Autodesk Fusion 360 part; units mm, degrees
(part 2 of 4)
extrude "Extrusion32" add sketch "Skizze34" along normal blind 12 contours L15 L31 L36 L66 L67 L68 L69 bodies 2
sketch "Skizze35" plane through (0, 47, 0) normal (0, 1, 0) x (-1, 0, 0)
  line L0 (23, -18.5) -> (23, -10.5)
  line L1 (23, -10.5) -> (30, -10.5)
  line L2 (30, -10.5) -> (30, -18.5)
  line L3 (30, -18.5) -> (23, -18.5)
  line L4 (21.5, -1.5) -> (21.5, -23.5)
  line L5 (21.5, -23.5) -> (-5.5, -23.5)
  line L6 (-5.5, -23.5) -> (-5.5, -1.5)
  line L7 (-5.5, -1.5) -> (21.5, -1.5)
  circle A0 centre (36, -25) radius 1.9
  circle A1 centre (-36, -14.5) radius 1.9
  circle A2 centre (36, 25) radius 1.9
  circle A3 centre (-36, 14.5) radius 1.9
  line L8 (-12, 21.5) -> (-12, 11.5)
  line L9 (-12, 11.5) -> (-21, 11.5)
  line L10 (-21, 11.5) -> (-21, 21.5)
  line L11 (-21, 21.5) -> (-22.5, 21.5)
  line L12 (-22.5, 21.5) -> (-22.5, 27.5)
  line L13 (-22.5, 27.5) -> (-32.5, 27.5)
  line L14 (-32.5, 27.5) -> (-32.5, 19)
  arc A4 (-33.5, 18) -> (-32.5, 19) centre (-33.5, 19) ccw
  line L15 (-33.5, 18) -> (-38.5, 18)
  arc A5 (-38.5, 18) -> (-39.5, 17) centre (-38.5, 17) ccw
  line L16 (-39.5, 17) -> (-39.5, 12)
  arc A6 (-40.5, 11) -> (-39.5, 12) centre (-40.5, 12) ccw
  line L17 (-40.5, 11) -> (-56.5, 11)
  line L18 (-56.5, 11) -> (-56.5, -11)
  line L19 (-56.5, -11) -> (-40.5, -11)
  arc A7 (-39.5, -12) -> (-40.5, -11) centre (-40.5, -12) ccw
  line L20 (-39.5, -12) -> (-39.5, -17)
  arc A8 (-39.5, -17) -> (-38.5, -18) centre (-38.5, -17) ccw
  line L21 (-38.5, -18) -> (-33.5, -18)
  arc A9 (-32.5, -19) -> (-33.5, -18) centre (-33.5, -19) ccw
  line L22 (-32.5, -19) -> (-32.5, -27.5)
  line L23 (-32.5, -27.5) -> (32.5, -27.5)
  line L24 (32.5, -27.5) -> (34.8649, -28.3108)
  arc A10 (34.8649, -28.3108) -> (38.922, -26.9266) centre (36, -25) ccw
  line L25 (38.922, -26.9266) -> (42.5, -21.5)
  line L26 (42.5, -21.5) -> (57.5, -6.5)
  line L27 (57.5, -6.5) -> (57.5, 6.5)
  line L28 (57.5, 6.5) -> (42.5, 21.5)
  line L29 (42.5, 21.5) -> (38.922, 26.9266)
  arc A11 (38.922, 26.9266) -> (34.8649, 28.3108) centre (36, 25) ccw
  line L30 (34.8649, 28.3108) -> (32.5, 27.5)
  line L31 (32.5, 27.5) -> (-10.5, 27.5)
  line L32 (-10.5, 27.5) -> (-10.5, 21.5)
  line L33 (-10.5, 21.5) -> (-12, 21.5)
  circle A12 centre (3.5, 16) radius 6.5
  line L34 (-1.75, 0) -> (-22.5, 0)
  line L35 (45, 1.5) -> (34, 1.5)
  arc A13 (34, 1.5) -> (34, -1.5) centre (34, 0) ccw
  line L36 (34, -1.5) -> (45, -1.5)
  arc A14 (45, -1.5) -> (45, 1.5) centre (45, 0) ccw
  line L37 (45, 0) -> (34, 0) construction
  arc A15 (45, -13.5) -> (45, -10.5) centre (45, -12) ccw
  line L38 (34, -13.5) -> (45, -13.5)
  arc A16 (34, -10.5) -> (34, -13.5) centre (34, -12) ccw
  line L39 (45, -10.5) -> (34, -10.5)
  arc A17 (45, -7.5) -> (45, -4.5) centre (45, -6) ccw
  line L40 (34, -7.5) -> (45, -7.5)
  arc A18 (34, -4.5) -> (34, -7.5) centre (34, -6) ccw
  line L41 (45, -4.5) -> (34, -4.5)
  arc A19 (45, 4.5) -> (45, 7.5) centre (45, 6) ccw
  line L42 (34, 4.5) -> (45, 4.5)
  arc A20 (34, 7.5) -> (34, 4.5) centre (34, 6) ccw
  line L43 (45, 7.5) -> (34, 7.5)
  arc A21 (45, 10.5) -> (45, 13.5) centre (45, 12) ccw
  line L44 (34, 10.5) -> (45, 10.5)
  arc A22 (34, 13.5) -> (34, 10.5) centre (34, 12) ccw
  line L45 (45, 13.5) -> (34, 13.5)
  line L46 (-48.5, -1.5) -> (-37.3325, -1.5)
  arc A23 (-37.3325, -1.5) -> (-37.3325, 1.5) centre (-37.3325, 0) ccw
  line L47 (-37.3325, 1.5) -> (-48.5, 1.5)
  arc A24 (-48.5, 1.5) -> (-48.5, -1.5) centre (-48.5, 0) ccw
  line L48 (-48.5, 0) -> (-37.3325, 0) construction
  arc A25 (-37.3325, -7.5) -> (-37.3325, -4.5) centre (-37.3325, -6) ccw
  line L49 (-48.5, -7.5) -> (-37.3325, -7.5)
  line L50 (-37.3325, -4.5) -> (-48.5, -4.5)
  arc A26 (-48.5, -4.5) -> (-48.5, -7.5) centre (-48.5, -6) ccw
  arc A27 (-37.3325, 4.5) -> (-37.3325, 7.5) centre (-37.3325, 6) ccw
  line L51 (-48.5, 4.5) -> (-37.3325, 4.5)
  line L52 (-37.3325, 7.5) -> (-48.5, 7.5)
  arc A28 (-48.5, 7.5) -> (-48.5, 4.5) centre (-48.5, 6) ccw
  line L53 (-12.5, 8.9343) -> (-20.5, 8.9343)
  arc A29 (-20.5, 8.9343) -> (-20.5, 6.9343) centre (-20.5, 7.9343) ccw
  line L54 (-20.5, 6.9343) -> (-12.5, 6.9343)
  arc A30 (-12.5, 6.9343) -> (-12.5, 8.9343) centre (-12.5, 7.9343) ccw
  line L55 (-12.5, 7.9343) -> (-20.5, 7.9343) construction
  arc A31 (-12.5, 2.5057) -> (-12.5, 4.5057) centre (-12.5, 3.5057) ccw
  line L56 (-20.5, 2.5057) -> (-12.5, 2.5057)
  line L57 (-12.5, 4.5057) -> (-20.5, 4.5057)
  arc A32 (-20.5, 4.5057) -> (-20.5, 2.5057) centre (-20.5, 3.5057) ccw
  arc A33 (-12.5, -1.9228) -> (-12.5, 0.0772) centre (-12.5, -0.9228) ccw
  line L58 (-20.5, -1.9228) -> (-12.5, -1.9228)
  line L59 (-12.5, 0.0772) -> (-20.5, 0.0772)
  arc A34 (-20.5, 0.0772) -> (-20.5, -1.9228) centre (-20.5, -0.9228) ccw
  arc A35 (-12.5, -6.3514) -> (-12.5, -4.3514) centre (-12.5, -5.3514) ccw
  line L60 (-20.5, -6.3514) -> (-12.5, -6.3514)
  line L61 (-12.5, -4.3514) -> (-20.5, -4.3514)
  arc A36 (-20.5, -4.3514) -> (-20.5, -6.3514) centre (-20.5, -5.3514) ccw
  arc A37 (-12.5, -10.78) -> (-12.5, -8.78) centre (-12.5, -9.78) ccw
  line L62 (-20.5, -10.78) -> (-12.5, -10.78)
  line L63 (-12.5, -8.78) -> (-20.5, -8.78)
  arc A38 (-20.5, -8.78) -> (-20.5, -10.78) centre (-20.5, -9.78) ccw
  arc A39 (-12.5, -15.2086) -> (-12.5, -13.2086) centre (-12.5, -14.2086) ccw
  line L64 (-20.5, -15.2086) -> (-12.5, -15.2086)
  line L65 (-12.5, -13.2086) -> (-20.5, -13.2086)
  arc A40 (-20.5, -13.2086) -> (-20.5, -15.2086) centre (-20.5, -14.2086) ccw
  arc A41 (-12.5, -19.6371) -> (-12.5, -17.6371) centre (-12.5, -18.6371) ccw
  line L66 (-20.5, -19.6371) -> (-12.5, -19.6371)
  line L67 (-12.5, -17.6371) -> (-20.5, -17.6371)
  arc A42 (-20.5, -17.6371) -> (-20.5, -19.6371) centre (-20.5, -18.6371) ccw
  arc A43 (-12.5, -24.0657) -> (-12.5, -22.0657) centre (-12.5, -23.0657) ccw
  line L68 (-20.5, -24.0657) -> (-12.5, -24.0657)
  line L69 (-12.5, -22.0657) -> (-20.5, -22.0657)
  arc A44 (-20.5, -22.0657) -> (-20.5, -24.0657) centre (-20.5, -23.0657) ccw
  dimension "d166" = 3
  dimension "d169" = 0
  dimension "d170" = 12
  dimension "d171" = 3
  dimension "d174" = 0
  dimension "d175" = 6
  dimension "d176" = 2
  dimension "d179" = 0
  dimension "d180" = -31
  measures "d166" diameter of A13
  measures "d171" diameter of A23
  measures "d176" diameter of A29
extrude "Extrusion33" cut sketch "Skizze35" against normal blind 2 contours L34 A33 L58 A34 | L35 A13 L36 A14 | A15 L38 A16 L39 | A17 L40 A18 L41 | A19 L42 A20 L43 | A21 L44 A22 L45 | L46 A23 L47 A24 | A25 L49 L50 A26 | A27 L51 L52 A28 | L53 A29 L54 A30 | A31 L56 L57 A32 | A35 L60 L61 A36 | A37 L62 L63 A38 | A39 L64 L65 A40 | A41 L66 L67 A42 | A43 L68 L69 A44 bodies 2
sketch "Skizze37" plane through (0, 45, 0) normal (0, -1, 0) x (1, 0, 0)
  line L0 (48.5, -7.5) -> (37.3325, -7.5)
  arc A0 (37.3325, -4.5) -> (37.3325, -7.5) centre (37.3325, -6) ccw
  line L1 (37.3325, -4.5) -> (48.5, -4.5)
  arc A1 (48.5, -7.5) -> (48.5, -4.5) centre (48.5, -6) ccw
  line L2 (20.5, -6.3514) -> (12.5, -6.3514)
  arc A2 (12.5, -4.3514) -> (12.5, -6.3514) centre (12.5, -5.3514) ccw
  line L3 (12.5, -4.3514) -> (20.5, -4.3514)
  arc A3 (20.5, -6.3514) -> (20.5, -4.3514) centre (20.5, -5.3514) ccw
  line L4 (20.5, -24.0657) -> (12.5, -24.0657)
  arc A4 (12.5, -22.0657) -> (12.5, -24.0657) centre (12.5, -23.0657) ccw
  line L5 (12.5, -22.0657) -> (20.5, -22.0657)
  arc A5 (20.5, -24.0657) -> (20.5, -22.0657) centre (20.5, -23.0657) ccw
  arc A6 (-34, -7.5) -> (-34, -4.5) centre (-34, -6) ccw
  line L6 (-34, -7.5) -> (-45, -7.5)
  arc A7 (-45, -4.5) -> (-45, -7.5) centre (-45, -6) ccw
  line L7 (-45, -4.5) -> (-34, -4.5)
  line L8 (-45, 1.5) -> (-34, 1.5)
  arc A8 (-34, -1.5) -> (-34, 1.5) centre (-34, 0) ccw
  line L9 (-34, -1.5) -> (-45, -1.5)
  arc A9 (-45, 1.5) -> (-45, -1.5) centre (-45, 0) ccw
  line L10 (20.5, -19.6371) -> (12.5, -19.6371)
  arc A10 (12.5, -17.6371) -> (12.5, -19.6371) centre (12.5, -18.6371) ccw
  line L11 (12.5, -17.6371) -> (20.5, -17.6371)
  arc A11 (20.5, -19.6371) -> (20.5, -17.6371) centre (20.5, -18.6371) ccw
  arc A12 (20.5, -1.9228) -> (20.8852, 0) centre (20.5, -0.9228) ccw
  line L12 (20.5, -1.9228) -> (12.5, -1.9228)
  arc A13 (12.1148, 0) -> (12.5, -1.9228) centre (12.5, -0.9228) ccw
  line L13 (12.1148, 0) -> (20.8852, 0)
  line L14 (48.5, -1.5) -> (37.3325, -1.5)
  arc A14 (37.3325, 1.5) -> (37.3325, -1.5) centre (37.3325, 0) ccw
  line L15 (37.3325, 1.5) -> (48.5, 1.5)
  arc A15 (48.5, -1.5) -> (48.5, 1.5) centre (48.5, 0) ccw
  line L16 (12.5, 8.9343) -> (20.5, 8.9343)
  arc A16 (20.5, 6.9343) -> (20.5, 8.9343) centre (20.5, 7.9343) ccw
  line L17 (20.5, 6.9343) -> (12.5, 6.9343)
  arc A17 (12.5, 8.9343) -> (12.5, 6.9343) centre (12.5, 7.9343) ccw
  line L18 (20.5, -10.78) -> (12.5, -10.78)
  arc A18 (12.5, -8.78) -> (12.5, -10.78) centre (12.5, -9.78) ccw
  line L19 (12.5, -8.78) -> (20.5, -8.78)
  arc A19 (20.5, -10.78) -> (20.5, -8.78) centre (20.5, -9.78) ccw
  arc A20 (-34, 10.5) -> (-34, 13.5) centre (-34, 12) ccw
  line L20 (-34, 10.5) -> (-45, 10.5)
  arc A21 (-45, 13.5) -> (-45, 10.5) centre (-45, 12) ccw
  line L21 (-45, 13.5) -> (-34, 13.5)
  arc A22 (-34, -13.5) -> (-34, -10.5) centre (-34, -12) ccw
  line L22 (-34, -13.5) -> (-45, -13.5)
  arc A23 (-45, -10.5) -> (-45, -13.5) centre (-45, -12) ccw
  line L23 (-45, -10.5) -> (-34, -10.5)
  arc A24 (-34, 4.5) -> (-34, 7.5) centre (-34, 6) ccw
  line L24 (-34, 4.5) -> (-45, 4.5)
  arc A25 (-45, 7.5) -> (-45, 4.5) centre (-45, 6) ccw
  line L25 (-45, 7.5) -> (-34, 7.5)
  line L26 (20.5, -15.2086) -> (12.5, -15.2086)
  arc A26 (12.5, -13.2086) -> (12.5, -15.2086) centre (12.5, -14.2086) ccw
  line L27 (12.5, -13.2086) -> (20.5, -13.2086)
  arc A27 (20.5, -15.2086) -> (20.5, -13.2086) centre (20.5, -14.2086) ccw
  line L28 (20.5, 2.5057) -> (12.5, 2.5057)
  arc A28 (12.5, 4.5057) -> (12.5, 2.5057) centre (12.5, 3.5057) ccw
  line L29 (12.5, 4.5057) -> (20.5, 4.5057)
  arc A29 (20.5, 2.5057) -> (20.5, 4.5057) centre (20.5, 3.5057) ccw
  line L30 (48.5, 4.5) -> (37.3325, 4.5)
  arc A30 (37.3325, 7.5) -> (37.3325, 4.5) centre (37.3325, 6) ccw
  line L31 (37.3325, 7.5) -> (48.5, 7.5)
  arc A31 (48.5, 4.5) -> (48.5, 7.5) centre (48.5, 6) ccw
  line L32 (-21.5, -20) -> (-31, -20)
  line L33 (-31, -20) -> (-31, -26)
  line L34 (-31, -26) -> (-23, -26)
  line L35 (-23, -26) -> (23, -26)
  line L36 (23, -26) -> (31, -26)
  line L37 (31, -26) -> (31, -9.5)
  line L38 (31, -9.5) -> (51.5, -9.5)
  line L39 (51.5, -9.5) -> (51.5, 9.5)
  line L40 (51.5, 9.5) -> (31, 9.5)
  line L41 (31, 9.5) -> (31, 26)
  line L42 (31, 26) -> (22.5, 26)
  line L43 (22.5, 26) -> (22.5, 21.5)
  line L44 (22.5, 21.5) -> (21, 21.5)
  line L45 (21, 21.5) -> (21, 11.5)
  line L46 (21, 11.5) -> (12, 11.5)
  line L47 (12, 11.5) -> (12, 21.5)
  line L48 (12, 21.5) -> (10.5, 21.5)
  line L49 (10.5, 21.5) -> (10.5, 26)
  line L50 (10.5, 26) -> (-31, 26)
  line L51 (-31, 26) -> (-31, 20)
  line L52 (-31, 20) -> (-41.8787, 20)
  line L53 (-41.8787, 20) -> (-51.5218, 10.3569)
  line L54 (-51.5218, 10.3569) -> (-51.5218, -10.3569)
  line L55 (-51.5218, -10.3569) -> (-41.8787, -20)
  line L56 (-41.8787, -20) -> (-31.5, -20)
  line L57 (-31.5, -20) -> (-31.5, -9)
  line L58 (-31.5, -9) -> (-21.5, -9)
  line L59 (-21.5, -9) -> (-21.5, -4.5)
  line L60 (-21.5, -4.5) -> (5.5, -4.5)
  line L61 (5.5, -4.5) -> (5.5, -20.5)
  line L62 (5.5, -20.5) -> (-21.5, -20.5)
  line L63 (-21.5, -20.5) -> (-21.5, -20)
  circle A32 centre (-3.5, 16) radius 6.5
  line L64 (26, -25.5) -> (8, -25.5)
  line L65 (8, -25.5) -> (8, 10.5)
  line L66 (8, 10.5) -> (26, 10.5)
  line L67 (26, 10.5) -> (26, -25.5)
  dimension "d185" = 18
  dimension "d186" = 36
  dimension "d187" = 8
  dimension "d188" = 5
  dimension "d189" = 1
  measures "d185" distance of origin
  measures "d186" distance of origin
  measures "d188" distance of L45 L67
  measures "d189" distance of L46 L66
extrude "Extrusion35" cut sketch "Skizze37" against normal blind 1 contours L64 L65 L66 L67 bodies 2
sketch "Skizze38" plane through (0, 47, 0) normal (0, 1, 0) x (-1, 0, 0)
  line L0 (-37.3325, -7.5) -> (-48.5, -7.5)
  arc A0 (-48.5, -4.5) -> (-48.5, -7.5) centre (-48.5, -6) ccw
  line L1 (-48.5, -4.5) -> (-37.3325, -4.5)
  arc A1 (-37.3325, -7.5) -> (-37.3325, -4.5) centre (-37.3325, -6) ccw
  line L2 (-12.5, -6.3514) -> (-20.5, -6.3514)
  arc A2 (-20.5, -4.3514) -> (-20.5, -6.3514) centre (-20.5, -5.3514) ccw
  line L3 (-20.5, -4.3514) -> (-12.5, -4.3514)
  arc A3 (-12.5, -6.3514) -> (-12.5, -4.3514) centre (-12.5, -5.3514) ccw
  line L4 (-12.5, -24.0657) -> (-20.5, -24.0657)
  arc A4 (-20.5, -22.0657) -> (-20.5, -24.0657) centre (-20.5, -23.0657) ccw
  line L5 (-20.5, -22.0657) -> (-12.5, -22.0657)
  arc A5 (-12.5, -24.0657) -> (-12.5, -22.0657) centre (-12.5, -23.0657) ccw
  arc A6 (34, -4.5) -> (34, -7.5) centre (34, -6) ccw
  line L6 (34, -4.5) -> (45, -4.5)
  arc A7 (45, -7.5) -> (45, -4.5) centre (45, -6) ccw
  line L7 (45, -7.5) -> (34, -7.5)
  line L8 (34, 1.5) -> (45, 1.5)
  arc A8 (45, -1.5) -> (45, 1.5) centre (45, 0) ccw
  line L9 (45, -1.5) -> (34, -1.5)
  arc A9 (34, 1.5) -> (34, -1.5) centre (34, 0) ccw
  line L10 (-12.5, -19.6371) -> (-20.5, -19.6371)
  arc A10 (-20.5, -17.6371) -> (-20.5, -19.6371) centre (-20.5, -18.6371) ccw
  line L11 (-20.5, -17.6371) -> (-12.5, -17.6371)
  arc A11 (-12.5, -19.6371) -> (-12.5, -17.6371) centre (-12.5, -18.6371) ccw
  arc A12 (-20.8852, 0) -> (-20.5, -1.9228) centre (-20.5, -0.9228) ccw
  line L12 (-20.8852, 0) -> (-12.1148, 0)
  arc A13 (-12.5, -1.9228) -> (-12.1148, 0) centre (-12.5, -0.9228) ccw
  line L13 (-12.5, -1.9228) -> (-20.5, -1.9228)
  line L14 (-37.3325, -1.5) -> (-48.5, -1.5)
  arc A14 (-48.5, 1.5) -> (-48.5, -1.5) centre (-48.5, 0) ccw
  line L15 (-48.5, 1.5) -> (-37.3325, 1.5)
  arc A15 (-37.3325, -1.5) -> (-37.3325, 1.5) centre (-37.3325, 0) ccw
  line L16 (-20.5, 8.9343) -> (-12.5, 8.9343)
  arc A16 (-12.5, 6.9343) -> (-12.5, 8.9343) centre (-12.5, 7.9343) ccw
  line L17 (-12.5, 6.9343) -> (-20.5, 6.9343)
  arc A17 (-20.5, 8.9343) -> (-20.5, 6.9343) centre (-20.5, 7.9343) ccw
  line L18 (-12.5, -10.78) -> (-20.5, -10.78)
  arc A18 (-20.5, -8.78) -> (-20.5, -10.78) centre (-20.5, -9.78) ccw
  line L19 (-20.5, -8.78) -> (-12.5, -8.78)
  arc A19 (-12.5, -10.78) -> (-12.5, -8.78) centre (-12.5, -9.78) ccw
  arc A20 (34, 13.5) -> (34, 10.5) centre (34, 12) ccw
  line L20 (34, 13.5) -> (45, 13.5)
  arc A21 (45, 10.5) -> (45, 13.5) centre (45, 12) ccw
  line L21 (45, 10.5) -> (34, 10.5)
  arc A22 (34, -10.5) -> (34, -13.5) centre (34, -12) ccw
  line L22 (34, -10.5) -> (45, -10.5)
  arc A23 (45, -13.5) -> (45, -10.5) centre (45, -12) ccw
  line L23 (45, -13.5) -> (34, -13.5)
  arc A24 (34, 7.5) -> (34, 4.5) centre (34, 6) ccw
  line L24 (34, 7.5) -> (45, 7.5)
  arc A25 (45, 4.5) -> (45, 7.5) centre (45, 6) ccw
  line L25 (45, 4.5) -> (34, 4.5)
  line L26 (-12.5, -15.2086) -> (-20.5, -15.2086)
  arc A26 (-20.5, -13.2086) -> (-20.5, -15.2086) centre (-20.5, -14.2086) ccw
  line L27 (-20.5, -13.2086) -> (-12.5, -13.2086)
  arc A27 (-12.5, -15.2086) -> (-12.5, -13.2086) centre (-12.5, -14.2086) ccw
  line L28 (-12.5, 2.5057) -> (-20.5, 2.5057)
  arc A28 (-20.5, 4.5057) -> (-20.5, 2.5057) centre (-20.5, 3.5057) ccw
  line L29 (-20.5, 4.5057) -> (-12.5, 4.5057)
  arc A29 (-12.5, 2.5057) -> (-12.5, 4.5057) centre (-12.5, 3.5057) ccw
  line L30 (-37.3325, 4.5) -> (-48.5, 4.5)
  arc A30 (-48.5, 7.5) -> (-48.5, 4.5) centre (-48.5, 6) ccw
  line L31 (-48.5, 7.5) -> (-37.3325, 7.5)
  arc A31 (-37.3325, 4.5) -> (-37.3325, 7.5) centre (-37.3325, 6) ccw
  line L32 (23, -18.5) -> (23, -10.5)
  line L33 (23, -10.5) -> (30, -10.5)
  line L34 (30, -10.5) -> (30, -18.5)
  line L35 (30, -18.5) -> (23, -18.5)
  line L36 (21.5, -1.5) -> (21.5, -23.5)
  line L37 (21.5, -23.5) -> (-5.5, -23.5)
  line L38 (-5.5, -23.5) -> (-5.5, -1.5)
  line L39 (-5.5, -1.5) -> (21.5, -1.5)
  circle A32 centre (-36, 14.5) radius 1.9
  circle A33 centre (36, 25) radius 1.9
  circle A34 centre (36, -25) radius 1.9
  circle A35 centre (-36, -14.5) radius 1.9
  line L40 (-12, 21.5) -> (-12, 11.5)
  line L41 (-12, 11.5) -> (-21, 11.5)
  line L42 (-21, 11.5) -> (-21, 21.5)
  line L43 (-21, 21.5) -> (-22.5, 21.5)
  line L44 (-22.5, 21.5) -> (-22.5, 27.5)
  line L45 (-22.5, 27.5) -> (-32.5, 27.5)
  line L46 (-32.5, 27.5) -> (-32.5, 19)
  arc A36 (-33.5, 18) -> (-32.5, 19) centre (-33.5, 19) ccw
  line L47 (-33.5, 18) -> (-38.5, 18)
  arc A37 (-38.5, 18) -> (-39.5, 17) centre (-38.5, 17) ccw
  line L48 (-39.5, 17) -> (-39.5, 12)
  arc A38 (-40.5, 11) -> (-39.5, 12) centre (-40.5, 12) ccw
  line L49 (-40.5, 11) -> (-56.5, 11)
  line L50 (-56.5, 11) -> (-56.5, -11)
  line L51 (-56.5, -11) -> (-40.5, -11)
  arc A39 (-39.5, -12) -> (-40.5, -11) centre (-40.5, -12) ccw
  line L52 (-39.5, -12) -> (-39.5, -17)
  arc A40 (-39.5, -17) -> (-38.5, -18) centre (-38.5, -17) ccw
  line L53 (-38.5, -18) -> (-33.5, -18)
  arc A41 (-32.5, -19) -> (-33.5, -18) centre (-33.5, -19) ccw
  line L54 (-32.5, -19) -> (-32.5, -27.5)
  line L55 (-32.5, -27.5) -> (32.5, -27.5)
  line L56 (32.5, -27.5) -> (34.8649, -28.3108)
  arc A42 (34.8649, -28.3108) -> (38.922, -26.9266) centre (36, -25) ccw
  line L57 (38.922, -26.9266) -> (42.5, -21.5)
  line L58 (42.5, -21.5) -> (57.5, -6.5)
  line L59 (57.5, -6.5) -> (57.5, 6.5)
  line L60 (57.5, 6.5) -> (42.5, 21.5)
  line L61 (42.5, 21.5) -> (38.922, 26.9266)
  arc A43 (38.922, 26.9266) -> (34.8649, 28.3108) centre (36, 25) ccw
  line L62 (34.8649, 28.3108) -> (32.5, 27.5)
  line L63 (32.5, 27.5) -> (-10.5, 27.5)
  line L64 (-10.5, 27.5) -> (-10.5, 21.5)
  line L65 (-10.5, 21.5) -> (-12, 21.5)
  circle A44 centre (3.5, 16) radius 6.5
  line L66 (23, -18.5) -> (22.3, -18.5)
  line L67 (22.3, -18.5) -> (22.3, -10.5)
  line L68 (22.3, -10.5) -> (23, -10.5)
  line L69 (23, -10.5) -> (23, -18.5)
  dimension "d192" = 0.7
  dimension "d194" = 0.8
  measures "d194" distance of L36 L67
extrude "Extrusion36" cut sketch "Skizze38" against normal blind 14 contours L32 L66 L67 L68 L69 bodies 2
sketch "Skizze39" plane through (0, 0, 0) normal (0, -1, 0) x (1, 0, 0)
  circle A0 centre (36, 14.5) radius 1.9
  circle A1 centre (36, -14.5) radius 1.9
  circle A2 centre (-36, -25) radius 1.9
  circle A3 centre (-36, 25) radius 1.9
  arc A4 (38.5, -18) -> (39.5, -17) centre (38.5, -17) ccw
  line L0 (39.5, -17) -> (39.5, -12)
  arc A5 (40.5, -11) -> (39.5, -12) centre (40.5, -12) ccw
  line L1 (40.5, -11) -> (56.5, -11)
  line L2 (56.5, -11) -> (56.5, 11)
  line L3 (56.5, 11) -> (40.5, 11)
  arc A6 (39.5, 12) -> (40.5, 11) centre (40.5, 12) ccw
  line L4 (39.5, 12) -> (39.5, 17)
  arc A7 (39.5, 17) -> (38.5, 18) centre (38.5, 17) ccw
  line L5 (38.5, 18) -> (33.5, 18)
  arc A8 (32.5, 19) -> (33.5, 18) centre (33.5, 19) ccw
  line L6 (32.5, 19) -> (32.5, 27.5)
  line L7 (32.5, 27.5) -> (-32.5, 27.5)
  line L8 (-32.5, 27.5) -> (-34.8649, 28.3108)
  arc A9 (-34.8649, 28.3108) -> (-38.922, 26.9266) centre (-36, 25) ccw
  line L9 (-38.922, 26.9266) -> (-42.5, 21.5)
  line L10 (-42.5, 21.5) -> (-57.5, 6.5)
  line L11 (-57.5, 6.5) -> (-57.5, -6.5)
  line L12 (-57.5, -6.5) -> (-42.5, -21.5)
  line L13 (-42.5, -21.5) -> (-38.922, -26.9266)
  arc A10 (-38.922, -26.9266) -> (-34.8649, -28.3108) centre (-36, -25) ccw
  line L14 (-34.8649, -28.3108) -> (-32.5, -27.5)
  line L15 (-32.5, -27.5) -> (32.5, -27.5)
  line L16 (32.5, -27.5) -> (32.5, -19)
  arc A11 (33.5, -18) -> (32.5, -19) centre (33.5, -19) ccw
  line L17 (33.5, -18) -> (38.5, -18)
  line L18 (31, -19) -> (32.5, -19)
  line L19 (32.5, -19) -> (32.5, -27.5)
  line L20 (32.5, -27.5) -> (-32.5, -27.5)
  line L21 (-32.5, -27.5) -> (-34.8649, -28.3108)
  arc A12 (-38.922, -26.9266) -> (-34.8649, -28.3108) centre (-36, -25) ccw
  line L22 (-38.922, -26.9266) -> (-42.5, -21.5)
  line L23 (-42.5, -21.5) -> (-57.5, -6.5)
  line L24 (-57.5, -6.5) -> (-57.5, -5)
  line L25 (-57.5, -5) -> (-51.5218, -5)
  line L26 (-51.5218, -5) -> (-51.5218, -10.3569)
  line L27 (-51.5218, -10.3569) -> (-41.8787, -20)
  line L28 (-41.8787, -20) -> (-31, -20)
  line L29 (-31, -20) -> (-31, -26)
  line L30 (-31, -26) -> (31, -26)
  line L31 (31, -26) -> (31, -19)
  circle A13 centre (-36, -25) radius 1.9
  circle A14 centre (-36, 25) radius 1.9
  line L32 (32.5, 19) -> (31, 19)
  line L33 (31, 19) -> (31, 26)
  line L34 (31, 26) -> (-31, 26)
  line L35 (-31, 26) -> (-31, 20)
  line L36 (-31, 20) -> (-41.8787, 20)
  line L37 (-41.8787, 20) -> (-51.5218, 10.3569)
  line L38 (-51.5218, 10.3569) -> (-51.5218, 5)
  line L39 (-51.5218, 5) -> (-57.5, 5)
  line L40 (-57.5, 5) -> (-57.5, 6.5)
  line L41 (-57.5, 6.5) -> (-42.5, 21.5)
  line L42 (-42.5, 21.5) -> (-38.922, 26.9266)
  arc A15 (-34.8649, 28.3108) -> (-38.922, 26.9266) centre (-36, 25) ccw
  line L43 (-34.8649, 28.3108) -> (-32.5, 27.5)
  line L44 (-32.5, 27.5) -> (32.5, 27.5)
  line L45 (32.5, 27.5) -> (32.5, 19)
  line L46 (51.5, -5) -> (56.5, -5)
  line L47 (56.5, -5) -> (56.5, -11)
  line L48 (56.5, -11) -> (40.5, -11)
  arc A16 (40.5, -11) -> (39.5, -12) centre (40.5, -12) ccw
  line L49 (39.5, -12) -> (39.5, -17)
  arc A17 (38.5, -18) -> (39.5, -17) centre (38.5, -17) ccw
  line L50 (38.5, -18) -> (33.5, -18)
  arc A18 (33.5, -18) -> (32.5, -19) centre (33.5, -19) ccw
  line L51 (32.5, -19) -> (31, -19)
  line L52 (31, -19) -> (31, -9.5)
  line L53 (31, -9.5) -> (51.5, -9.5)
  line L54 (51.5, -9.5) -> (51.5, -5)
  circle A19 centre (36, -14.5) radius 1.9
  line L55 (56.5, 5) -> (51.5, 5)
  line L56 (51.5, 5) -> (51.5, 9.5)
  line L57 (51.5, 9.5) -> (31, 9.5)
  line L58 (31, 9.5) -> (31, 19)
  line L59 (31, 19) -> (32.5, 19)
  arc A20 (32.5, 19) -> (33.5, 18) centre (33.5, 19) ccw
  line L60 (33.5, 18) -> (38.5, 18)
  arc A21 (39.5, 17) -> (38.5, 18) centre (38.5, 17) ccw
  line L61 (39.5, 17) -> (39.5, 12)
  arc A22 (39.5, 12) -> (40.5, 11) centre (40.5, 12) ccw
  line L62 (40.5, 11) -> (56.5, 11)
  line L63 (56.5, 11) -> (56.5, 5)
  circle A23 centre (36, 14.5) radius 1.9
  line L64 (-37.5877, -22.25) -> (-39.1754, -25)
  line L65 (-39.1754, -25) -> (-37.5877, -27.75)
  line L66 (-37.5877, -27.75) -> (-34.4123, -27.75)
  line L67 (-34.4123, -27.75) -> (-32.8246, -25)
  line L68 (-32.8246, -25) -> (-34.4123, -22.25)
  line L69 (-34.4123, -22.25) -> (-37.5877, -22.25)
  line L70 (-34.4123, 22.25) -> (-32.8246, 25)
  line L71 (-32.8246, 25) -> (-34.4123, 27.75)
  line L72 (-34.4123, 27.75) -> (-37.5877, 27.75)
  line L73 (-37.5877, 27.75) -> (-39.1754, 25)
  line L74 (-39.1754, 25) -> (-37.5877, 22.25)
  line L75 (-37.5877, 22.25) -> (-34.4123, 22.25)
  line L76 (34.4123, 17.25) -> (32.8246, 14.5)
  line L77 (32.8246, 14.5) -> (34.4123, 11.75)
  line L78 (34.4123, 11.75) -> (37.5877, 11.75)
  line L79 (37.5877, 11.75) -> (39.1754, 14.5)
  line L80 (39.1754, 14.5) -> (37.5877, 17.25)
  line L81 (37.5877, 17.25) -> (34.4123, 17.25)
  line L82 (34.4123, -11.75) -> (32.8246, -14.5)
  line L83 (32.8246, -14.5) -> (34.4123, -17.25)
  line L84 (34.4123, -17.25) -> (37.5877, -17.25)
  line L85 (37.5877, -17.25) -> (39.1754, -14.5)
  line L86 (39.1754, -14.5) -> (37.5877, -11.75)
  line L87 (37.5877, -11.75) -> (34.4123, -11.75)
  dimension "d197" = 5.5
  dimension "d198" = 5.5
  dimension "d199" = 5.5
  dimension "d200" = 5.5
  measures "d197" distance of L66 L69
  measures "d198" distance of L72 L75
  measures "d199" distance of L84 L87
  measures "d200" distance of L78 L81
extrude "Extrusion37" cut sketch "Skizze39" against normal blind 3 contours L64 L65 L66 L67 L68 L69 | L70 L71 L72 L73 L74 L75 | L76 L77 L78 L79 L80 L81 | L82 L83 L84 L85 L86 L87 bodies 1
sketch "Skizze40" plane through (0, 0, 0) normal (0, -1, 0) x (1, 0, 0)
  line L0 (32.8246, 14.5) -> (34.4123, 17.25)
  line L1 (34.4123, 17.25) -> (37.5877, 17.25)
  line L2 (37.5877, 17.25) -> (39.1754, 14.5)
  line L3 (39.1754, 14.5) -> (37.5877, 11.75)
  line L4 (37.5877, 11.75) -> (34.4123, 11.75)
  line L5 (34.4123, 11.75) -> (32.8246, 14.5)
  line L6 (-32.8246, 25) -> (-34.4123, 22.25)
  line L7 (-34.4123, 22.25) -> (-37.5877, 22.25)
  line L8 (-37.5877, 22.25) -> (-39.1754, 25)
  line L9 (-39.1754, 25) -> (-37.5877, 27.75)
  line L10 (-37.5877, 27.75) -> (-34.4123, 27.75)
  line L11 (-34.4123, 27.75) -> (-32.8246, 25)
  line L12 (32.8246, -14.5) -> (34.4123, -11.75)
  line L13 (34.4123, -11.75) -> (37.5877, -11.75)
  line L14 (37.5877, -11.75) -> (39.1754, -14.5)
  line L15 (39.1754, -14.5) -> (37.5877, -17.25)
  line L16 (37.5877, -17.25) -> (34.4123, -17.25)
  line L17 (34.4123, -17.25) -> (32.8246, -14.5)
  line L18 (-39.1754, -25) -> (-37.5877, -22.25)
  line L19 (-37.5877, -22.25) -> (-34.4123, -22.25)
  line L20 (-34.4123, -22.25) -> (-32.8246, -25)
  line L21 (-32.8246, -25) -> (-34.4123, -27.75)
  line L22 (-34.4123, -27.75) -> (-37.5877, -27.75)
  line L23 (-37.5877, -27.75) -> (-39.1754, -25)
  arc A0 (38.5, -18) -> (39.5, -17) centre (38.5, -17) ccw
  line L24 (39.5, -17) -> (39.5, -12)
  arc A1 (40.5, -11) -> (39.5, -12) centre (40.5, -12) ccw
  line L25 (40.5, -11) -> (56.5, -11)
  line L26 (56.5, -11) -> (56.5, 11)
  line L27 (56.5, 11) -> (40.5, 11)
  arc A2 (39.5, 12) -> (40.5, 11) centre (40.5, 12) ccw
  line L28 (39.5, 12) -> (39.5, 17)
  arc A3 (39.5, 17) -> (38.5, 18) centre (38.5, 17) ccw
  line L29 (38.5, 18) -> (33.5, 18)
  arc A4 (32.5, 19) -> (33.5, 18) centre (33.5, 19) ccw
  line L30 (32.5, 19) -> (32.5, 27.5)
  line L31 (32.5, 27.5) -> (-32.5, 27.5)
  line L32 (-32.5, 27.5) -> (-34.8649, 28.3108)
  arc A5 (-34.8649, 28.3108) -> (-38.922, 26.9266) centre (-36, 25) ccw
  line L33 (-38.922, 26.9266) -> (-42.5, 21.5)
  line L34 (-42.5, 21.5) -> (-57.5, 6.5)
  line L35 (-57.5, 6.5) -> (-57.5, -6.5)
  line L36 (-57.5, -6.5) -> (-42.5, -21.5)
  line L37 (-42.5, -21.5) -> (-38.922, -26.9266)
  arc A6 (-38.922, -26.9266) -> (-34.8649, -28.3108) centre (-36, -25) ccw
  line L38 (-34.8649, -28.3108) -> (-32.5, -27.5)
  line L39 (-32.5, -27.5) -> (32.5, -27.5)
  line L40 (32.5, -27.5) -> (32.5, -19)
  arc A7 (33.5, -18) -> (32.5, -19) centre (33.5, -19) ccw
  line L41 (33.5, -18) -> (38.5, -18)
  line L42 (31, -19) -> (32.5, -19)
  line L43 (32.5, -19) -> (32.5, -27.5)
  line L44 (32.5, -27.5) -> (-32.5, -27.5)
  line L45 (-32.5, -27.5) -> (-34.8649, -28.3108)
  arc A8 (-38.922, -26.9266) -> (-34.8649, -28.3108) centre (-36, -25) ccw
  line L46 (-38.922, -26.9266) -> (-42.5, -21.5)
  line L47 (-42.5, -21.5) -> (-57.5, -6.5)
  line L48 (-57.5, -6.5) -> (-57.5, -5)
  line L49 (-57.5, -5) -> (-51.5218, -5)
  line L50 (-51.5218, -5) -> (-51.5218, -10.3569)
  line L51 (-51.5218, -10.3569) -> (-41.8787, -20)
  line L52 (-41.8787, -20) -> (-31, -20)
  line L53 (-31, -20) -> (-31, -26)
  line L54 (-31, -26) -> (31, -26)
  line L55 (31, -26) -> (31, -19)
  circle A9 centre (-36, -25) radius 1.9
  circle A10 centre (-36, 25) radius 1.9
  line L56 (32.5, 19) -> (31, 19)
  line L57 (31, 19) -> (31, 26)
  line L58 (31, 26) -> (-31, 26)
  line L59 (-31, 26) -> (-31, 20)
  line L60 (-31, 20) -> (-41.8787, 20)
  line L61 (-41.8787, 20) -> (-51.5218, 10.3569)
  line L62 (-51.5218, 10.3569) -> (-51.5218, 5)
  line L63 (-51.5218, 5) -> (-57.5, 5)
  line L64 (-57.5, 5) -> (-57.5, 6.5)
  line L65 (-57.5, 6.5) -> (-42.5, 21.5)
  line L66 (-42.5, 21.5) -> (-38.922, 26.9266)
  arc A11 (-34.8649, 28.3108) -> (-38.922, 26.9266) centre (-36, 25) ccw
  line L67 (-34.8649, 28.3108) -> (-32.5, 27.5)
  line L68 (-32.5, 27.5) -> (32.5, 27.5)
  line L69 (32.5, 27.5) -> (32.5, 19)
  circle A12 centre (-36, -25) radius 4
  line L70 (-42.5, -21.5) -> (-39.5022, -26.9326)
  line L71 (-32.5, -27.5) -> (-33.8276, -28.3587)
  line L72 (1.75, 0) -> (22.5, 0)
  line L73 (-42.5, 21.5) -> (-39.5022, 26.9326)
  circle A13 centre (-36, 25) radius 4
  line L74 (-32.5, 27.5) -> (-33.8276, 28.3587)
  line L75 (51.5, -5) -> (56.5, -5)
  line L76 (56.5, -5) -> (56.5, -11)
  line L77 (56.5, -11) -> (40.5, -11)
  arc A14 (40.5, -11) -> (39.5, -12) centre (40.5, -12) ccw
  line L78 (39.5, -12) -> (39.5, -17)
  arc A15 (38.5, -18) -> (39.5, -17) centre (38.5, -17) ccw
  line L79 (38.5, -18) -> (33.5, -18)
  arc A16 (33.5, -18) -> (32.5, -19) centre (33.5, -19) ccw
  line L80 (32.5, -19) -> (31, -19)
  line L81 (31, -19) -> (31, -9.5)
  line L82 (31, -9.5) -> (51.5, -9.5)
  line L83 (51.5, -9.5) -> (51.5, -5)
  circle A17 centre (36, -14.5) radius 1.9
  line L84 (56.5, 5) -> (51.5, 5)
  line L85 (51.5, 5) -> (51.5, 9.5)
  line L86 (51.5, 9.5) -> (31, 9.5)
  line L87 (31, 9.5) -> (31, 19)
  line L88 (31, 19) -> (32.5, 19)
  arc A18 (32.5, 19) -> (33.5, 18) centre (33.5, 19) ccw
  line L89 (33.5, 18) -> (38.5, 18)
  arc A19 (39.5, 17) -> (38.5, 18) centre (38.5, 17) ccw
  line L90 (39.5, 17) -> (39.5, 12)
  arc A20 (39.5, 12) -> (40.5, 11) centre (40.5, 12) ccw
  line L91 (40.5, 11) -> (56.5, 11)
  line L92 (56.5, 11) -> (56.5, 5)
  circle A21 centre (36, 14.5) radius 1.9
  line L93 (38.5, -18) -> (40.5, -18)
  line L94 (40.5, -18) -> (40.5, -11)
  line L95 (40.5, -11) -> (38.5, -11)
  line L96 (38.5, -11) -> (38.5, -18)
  line L97 (38.5, 18) -> (40.5, 18)
  line L98 (40.5, 18) -> (40.5, 11)
  line L99 (40.5, 11) -> (38.5, 11)
  line L100 (38.5, 11) -> (38.5, 18)
  dimension "d203" = 8
  measures "d203" diameter of A12
extrude "Extrusion38" add sketch "Skizze40" against normal blind 16 contours A2 L28 A3 A19 L90 A20 L97 L98 | L32 L67 A13 L74 | L32 A5 L33 L66 A11 L67 A13 | L33 L66 L73 A13 | A0 L24 A1 A14 L78 A15 L93 L94 | L38 L45 A12 L71 | L37 L46 A12 L70 | L37 A6 L38 L45 A8 L46 A12 picked at (-38.4473, 27.9408) picked at (-38.4473, -27.9408) bodies 1
extrude "Extrusion39" add 2 faces at (40.1667, 16, -13.6667) (40.1667, 16, 15.3333) along direction (0, 1, 0) blind 5.5 on bodies 1 bodies 1
sketch "Skizze41" plane through (0, 47, 0) normal (0, 1, 0) x (-1, 0, 0)
  line L0 (22.3, -10.5) -> (30, -10.5)
  line L1 (30, -10.5) -> (30, -18.5)
  line L2 (30, -18.5) -> (22.3, -18.5)
  line L3 (22.3, -18.5) -> (22.3, -10.5)
  line L4 (-37.3325, -7.5) -> (-48.5, -7.5)
  arc A0 (-48.5, -4.5) -> (-48.5, -7.5) centre (-48.5, -6) ccw
  line L5 (-48.5, -4.5) -> (-37.3325, -4.5)
  arc A1 (-37.3325, -7.5) -> (-37.3325, -4.5) centre (-37.3325, -6) ccw
  line L6 (-12.5, -6.3514) -> (-20.5, -6.3514)
  arc A2 (-20.5, -4.3514) -> (-20.5, -6.3514) centre (-20.5, -5.3514) ccw
  line L7 (-20.5, -4.3514) -> (-12.5, -4.3514)
  arc A3 (-12.5, -6.3514) -> (-12.5, -4.3514) centre (-12.5, -5.3514) ccw
  line L8 (-12.5, -24.0657) -> (-20.5, -24.0657)
  arc A4 (-20.5, -22.0657) -> (-20.5, -24.0657) centre (-20.5, -23.0657) ccw
  line L9 (-20.5, -22.0657) -> (-12.5, -22.0657)
  arc A5 (-12.5, -24.0657) -> (-12.5, -22.0657) centre (-12.5, -23.0657) ccw
  arc A6 (34, -4.5) -> (34, -7.5) centre (34, -6) ccw
  line L10 (34, -4.5) -> (45, -4.5)
  arc A7 (45, -7.5) -> (45, -4.5) centre (45, -6) ccw
  line L11 (45, -7.5) -> (34, -7.5)
  line L12 (34, 1.5) -> (45, 1.5)
  arc A8 (45, -1.5) -> (45, 1.5) centre (45, 0) ccw
  line L13 (45, -1.5) -> (34, -1.5)
  arc A9 (34, 1.5) -> (34, -1.5) centre (34, 0) ccw
  line L14 (-12.5, -19.6371) -> (-20.5, -19.6371)
  arc A10 (-20.5, -17.6371) -> (-20.5, -19.6371) centre (-20.5, -18.6371) ccw
  line L15 (-20.5, -17.6371) -> (-12.5, -17.6371)
  arc A11 (-12.5, -19.6371) -> (-12.5, -17.6371) centre (-12.5, -18.6371) ccw
  arc A12 (-20.8852, 0) -> (-20.5, -1.9228) centre (-20.5, -0.9228) ccw
  line L16 (-20.8852, 0) -> (-12.1148, 0)
  arc A13 (-12.5, -1.9228) -> (-12.1148, 0) centre (-12.5, -0.9228) ccw
  line L17 (-12.5, -1.9228) -> (-20.5, -1.9228)
  line L18 (-37.3325, -1.5) -> (-48.5, -1.5)
  arc A14 (-48.5, 1.5) -> (-48.5, -1.5) centre (-48.5, 0) ccw
  line L19 (-48.5, 1.5) -> (-37.3325, 1.5)
  arc A15 (-37.3325, -1.5) -> (-37.3325, 1.5) centre (-37.3325, 0) ccw
  line L20 (-20.5, 8.9343) -> (-12.5, 8.9343)
  arc A16 (-12.5, 6.9343) -> (-12.5, 8.9343) centre (-12.5, 7.9343) ccw
  line L21 (-12.5, 6.9343) -> (-20.5, 6.9343)
  arc A17 (-20.5, 8.9343) -> (-20.5, 6.9343) centre (-20.5, 7.9343) ccw
  line L22 (-12.5, -10.78) -> (-20.5, -10.78)
  arc A18 (-20.5, -8.78) -> (-20.5, -10.78) centre (-20.5, -9.78) ccw
  line L23 (-20.5, -8.78) -> (-12.5, -8.78)
  arc A19 (-12.5, -10.78) -> (-12.5, -8.78) centre (-12.5, -9.78) ccw
  arc A20 (34, 13.5) -> (34, 10.5) centre (34, 12) ccw
  line L24 (34, 13.5) -> (45, 13.5)
  arc A21 (45, 10.5) -> (45, 13.5) centre (45, 12) ccw
  line L25 (45, 10.5) -> (34, 10.5)
  arc A22 (34, -10.5) -> (34, -13.5) centre (34, -12) ccw
  line L26 (34, -10.5) -> (45, -10.5)
  arc A23 (45, -13.5) -> (45, -10.5) centre (45, -12) ccw
  line L27 (45, -13.5) -> (34, -13.5)
  arc A24 (34, 7.5) -> (34, 4.5) centre (34, 6) ccw
  line L28 (34, 7.5) -> (45, 7.5)
  arc A25 (45, 4.5) -> (45, 7.5) centre (45, 6) ccw
  line L29 (45, 4.5) -> (34, 4.5)
  line L30 (-12.5, -15.2086) -> (-20.5, -15.2086)
  arc A26 (-20.5, -13.2086) -> (-20.5, -15.2086) centre (-20.5, -14.2086) ccw
  line L31 (-20.5, -13.2086) -> (-12.5, -13.2086)
  arc A27 (-12.5, -15.2086) -> (-12.5, -13.2086) centre (-12.5, -14.2086) ccw
  line L32 (-12.5, 2.5057) -> (-20.5, 2.5057)
  arc A28 (-20.5, 4.5057) -> (-20.5, 2.5057) centre (-20.5, 3.5057) ccw
  line L33 (-20.5, 4.5057) -> (-12.5, 4.5057)
  arc A29 (-12.5, 2.5057) -> (-12.5, 4.5057) centre (-12.5, 3.5057) ccw
  line L34 (-37.3325, 4.5) -> (-48.5, 4.5)
  arc A30 (-48.5, 7.5) -> (-48.5, 4.5) centre (-48.5, 6) ccw
  line L35 (-48.5, 7.5) -> (-37.3325, 7.5)
  arc A31 (-37.3325, 4.5) -> (-37.3325, 7.5) centre (-37.3325, 6) ccw
  line L36 (21.5, -1.5) -> (21.5, -23.5)
  line L37 (21.5, -23.5) -> (-5.5, -23.5)
  line L38 (-5.5, -23.5) -> (-5.5, -1.5)
  line L39 (-5.5, -1.5) -> (21.5, -1.5)
  circle A32 centre (-36, 14.5) radius 1.9
  circle A33 centre (36, 25) radius 1.9
  circle A34 centre (36, -25) radius 1.9
  circle A35 centre (-36, -14.5) radius 1.9
  line L40 (-12, 21.5) -> (-12, 11.5)
  line L41 (-12, 11.5) -> (-21, 11.5)
  line L42 (-21, 11.5) -> (-21, 21.5)
  line L43 (-21, 21.5) -> (-22.5, 21.5)
  line L44 (-22.5, 21.5) -> (-22.5, 27.5)
  line L45 (-22.5, 27.5) -> (-32.5, 27.5)
  line L46 (-32.5, 27.5) -> (-32.5, 19)
  arc A36 (-33.5, 18) -> (-32.5, 19) centre (-33.5, 19) ccw
  line L47 (-33.5, 18) -> (-38.5, 18)
  arc A37 (-38.5, 18) -> (-39.5, 17) centre (-38.5, 17) ccw
  line L48 (-39.5, 17) -> (-39.5, 12)
  arc A38 (-40.5, 11) -> (-39.5, 12) centre (-40.5, 12) ccw
  line L49 (-40.5, 11) -> (-56.5, 11)
  line L50 (-56.5, 11) -> (-56.5, -11)
  line L51 (-56.5, -11) -> (-40.5, -11)
  arc A39 (-39.5, -12) -> (-40.5, -11) centre (-40.5, -12) ccw
  line L52 (-39.5, -12) -> (-39.5, -17)
  arc A40 (-39.5, -17) -> (-38.5, -18) centre (-38.5, -17) ccw
  line L53 (-38.5, -18) -> (-33.5, -18)
  arc A41 (-32.5, -19) -> (-33.5, -18) centre (-33.5, -19) ccw
  line L54 (-32.5, -19) -> (-32.5, -27.5)
  line L55 (-32.5, -27.5) -> (32.5, -27.5)
  line L56 (32.5, -27.5) -> (34.8649, -28.3108)
  arc A42 (34.8649, -28.3108) -> (38.922, -26.9266) centre (36, -25) ccw
  line L57 (38.922, -26.9266) -> (42.5, -21.5)
  line L58 (42.5, -21.5) -> (57.5, -6.5)
  line L59 (57.5, -6.5) -> (57.5, 6.5)
  line L60 (57.5, 6.5) -> (42.5, 21.5)
  line L61 (42.5, 21.5) -> (38.922, 26.9266)
  arc A43 (38.922, 26.9266) -> (34.8649, 28.3108) centre (36, 25) ccw
  line L62 (34.8649, 28.3108) -> (32.5, 27.5)
  line L63 (32.5, 27.5) -> (-10.5, 27.5)
  line L64 (-10.5, 27.5) -> (-10.5, 21.5)
  line L65 (-10.5, 21.5) -> (-12, 21.5)
  circle A44 centre (3.5, 16) radius 6.5
  circle A45 centre (36, 25) radius 1.9
  line L66 (-32.5, 19) -> (-31, 19)
  line L67 (-31, 19) -> (-31, 26)
  line L68 (-31, 26) -> (31, 26)
  line L69 (31, 26) -> (31, 20)
  line L70 (31, 20) -> (41.8787, 20)
  line L71 (41.8787, 20) -> (51.5218, 10.3569)
  line L72 (51.5218, 10.3569) -> (51.5218, 5)
  line L73 (51.5218, 5) -> (57.5, 5)
  line L74 (57.5, 5) -> (57.5, 6.5)
  line L75 (57.5, 6.5) -> (42.5, 21.5)
  line L76 (42.5, 21.5) -> (39.5022, 26.9326)
  arc A46 (39.5022, 26.9326) -> (33.8276, 28.3587) centre (36, 25) ccw
  line L77 (33.8276, 28.3587) -> (32.5, 27.5)
  line L78 (32.5, 27.5) -> (-32.5, 27.5)
  line L79 (-32.5, 27.5) -> (-32.5, 19)
  line L80 (57.5, 5) -> (51.5218, 5)
  line L81 (51.5218, 5) -> (51.5218, 10.3569)
  line L82 (51.5218, 10.3569) -> (41.8787, 20)
  line L83 (41.8787, 20) -> (31, 20)
  line L84 (31, 20) -> (31, 26)
  line L85 (31, 26) -> (-31, 26)
  line L86 (-31, 26) -> (-31, 19)
  line L87 (-31, 19) -> (-32.5, 19)
  line L88 (-32.5, 19) -> (-32.5, 27.5)
  line L89 (-32.5, 27.5) -> (32.5, 27.5)
  line L90 (32.5, 27.5) -> (34.8649, 28.3108)
  arc A47 (38.922, 26.9266) -> (34.8649, 28.3108) centre (36, 25) ccw
  line L91 (38.922, 26.9266) -> (42.5, 21.5)
  line L92 (42.5, 21.5) -> (57.5, 6.5)
  line L93 (57.5, 6.5) -> (57.5, 5)
  circle A48 centre (36, 25) radius 1.9
  line L94 (-31, -19) -> (-32.5, -19)
  line L95 (-32.5, -19) -> (-32.5, -27.5)
  line L96 (-32.5, -27.5) -> (32.5, -27.5)
  line L97 (32.5, -27.5) -> (33.8276, -28.3587)
  arc A49 (33.8276, -28.3587) -> (39.5022, -26.9326) centre (36, -25) ccw
  line L98 (39.5022, -26.9326) -> (42.5, -21.5)
  line L99 (42.5, -21.5) -> (57.5, -6.5)
  line L100 (57.5, -6.5) -> (57.5, -5)
  line L101 (57.5, -5) -> (51.5218, -5)
  line L102 (51.5218, -5) -> (51.5218, -10.3569)
  line L103 (51.5218, -10.3569) -> (41.8787, -20)
  line L104 (41.8787, -20) -> (31, -20)
  line L105 (31, -20) -> (31, -26)
  line L106 (31, -26) -> (-31, -26)
  line L107 (-31, -26) -> (-31, -19)
  circle A50 centre (36, -25) radius 1.9
  line L108 (-32.8246, 14.5) -> (-34.4123, 17.25)
  line L109 (-34.4123, 17.25) -> (-37.5877, 17.25)
  line L110 (-37.5877, 17.25) -> (-39.1754, 14.5)
  line L111 (-39.1754, 14.5) -> (-37.5877, 11.75)
  line L112 (-37.5877, 11.75) -> (-34.4123, 11.75)
  line L113 (-34.4123, 11.75) -> (-32.8246, 14.5)
  line L114 (32.8246, 25) -> (34.4123, 22.25)
  line L115 (34.4123, 22.25) -> (37.5877, 22.25)
  line L116 (37.5877, 22.25) -> (39.1754, 25)
  line L117 (39.1754, 25) -> (37.5877, 27.75)
  line L118 (37.5877, 27.75) -> (34.4123, 27.75)
  line L119 (34.4123, 27.75) -> (32.8246, 25)
  line L120 (-32.8246, -14.5) -> (-34.4123, -11.75)
  line L121 (-34.4123, -11.75) -> (-37.5877, -11.75)
  line L122 (-37.5877, -11.75) -> (-39.1754, -14.5)
  line L123 (-39.1754, -14.5) -> (-37.5877, -17.25)
  line L124 (-37.5877, -17.25) -> (-34.4123, -17.25)
  line L125 (-34.4123, -17.25) -> (-32.8246, -14.5)
  line L126 (39.1754, -25) -> (37.5877, -22.25)
  line L127 (37.5877, -22.25) -> (34.4123, -22.25)
  line L128 (34.4123, -22.25) -> (32.8246, -25)
  line L129 (32.8246, -25) -> (34.4123, -27.75)
  line L130 (34.4123, -27.75) -> (37.5877, -27.75)
  line L131 (37.5877, -27.75) -> (39.1754, -25)
  line L132 (-40.5, -11) -> (-56.5, -11)
  line L133 (-56.5, -11) -> (-56.5, 11)
  line L134 (-56.5, 11) -> (-40.5, 11)
  line L135 (-40.5, 11) -> (-40.5, 18)
  line L136 (-40.5, 18) -> (-33.5, 18)
  arc A51 (-33.5, 18) -> (-32.5, 19) centre (-33.5, 19) ccw
  line L137 (-32.5, 19) -> (-32.5, 27.5)
  line L138 (-32.5, 27.5) -> (32.5, 27.5)
  line L139 (32.5, 27.5) -> (33.8276, 28.3587)
  arc A52 (39.5022, 26.9326) -> (33.8276, 28.3587) centre (36, 25) ccw
  line L140 (39.5022, 26.9326) -> (42.5, 21.5)
  line L141 (42.5, 21.5) -> (57.5, 6.5)
  line L142 (57.5, 6.5) -> (57.5, -6.5)
  line L143 (57.5, -6.5) -> (42.5, -21.5)
  line L144 (42.5, -21.5) -> (39.5022, -26.9326)
  arc A53 (33.8276, -28.3587) -> (39.5022, -26.9326) centre (36, -25) ccw
  line L145 (33.8276, -28.3587) -> (32.5, -27.5)
  line L146 (32.5, -27.5) -> (-32.5, -27.5)
  line L147 (-32.5, -27.5) -> (-32.5, -19)
  arc A54 (-32.5, -19) -> (-33.5, -18) centre (-33.5, -19) ccw
  line L148 (-33.5, -18) -> (-40.5, -18)
  line L149 (-40.5, -18) -> (-40.5, -11)
  line L150 (-40.5, -18) -> (-33.5, -18)
  arc A55 (-32.5, -19) -> (-33.5, -18) centre (-33.5, -19) ccw
  line L151 (-32.5, -19) -> (-31, -19)
  line L152 (-31, -19) -> (-31, -9.5)
  line L153 (-31, -9.5) -> (-51.5, -9.5)
  line L154 (-51.5, -9.5) -> (-51.5, -5)
  line L155 (-51.5, -5) -> (-56.5, -5)
  line L156 (-56.5, -5) -> (-56.5, -11)
  line L157 (-56.5, -11) -> (-40.5, -11)
  line L158 (-40.5, -11) -> (-40.5, -18)
  circle A56 centre (-36, -14.5) radius 1.9
  line L159 (-56.5, -5) -> (-51.5, -5)
  line L160 (-51.5, -5) -> (-51.5, -9.5)
  line L161 (-51.5, -9.5) -> (-31, -9.5)
  line L162 (-31, -9.5) -> (-31, -19)
  line L163 (-31, -19) -> (-32.5, -19)
  arc A57 (-32.5, -19) -> (-33.5, -18) centre (-33.5, -19) ccw
  line L164 (-33.5, -18) -> (-38.5, -18)
  arc A58 (-39.5, -17) -> (-38.5, -18) centre (-38.5, -17) ccw
  line L165 (-39.5, -17) -> (-39.5, -12)
  arc A59 (-39.5, -12) -> (-40.5, -11) centre (-40.5, -12) ccw
  line L166 (-40.5, -11) -> (-56.5, -11)
  line L167 (-56.5, -11) -> (-56.5, -5)
  circle A60 centre (-36, -14.5) radius 1.9
  line L168 (-56.5, 5) -> (-51.5, 5)
  line L169 (-51.5, 5) -> (-51.5, 9.5)
  line L170 (-51.5, 9.5) -> (-31, 9.5)
  line L171 (-31, 9.5) -> (-31, 19)
  line L172 (-31, 19) -> (-32.5, 19)
  arc A61 (-33.5, 18) -> (-32.5, 19) centre (-33.5, 19) ccw
  line L173 (-33.5, 18) -> (-40.5, 18)
  line L174 (-40.5, 18) -> (-40.5, 11)
  line L175 (-40.5, 11) -> (-56.5, 11)
  line L176 (-56.5, 11) -> (-56.5, 5)
  circle A62 centre (-36, 14.5) radius 1.9
  line L177 (-51.5, 5) -> (-56.5, 5)
  line L178 (-56.5, 5) -> (-56.5, 11)
  line L179 (-56.5, 11) -> (-40.5, 11)
  arc A63 (-40.5, 11) -> (-39.5, 12) centre (-40.5, 12) ccw
  line L180 (-39.5, 12) -> (-39.5, 17)
  arc A64 (-38.5, 18) -> (-39.5, 17) centre (-38.5, 17) ccw
  line L181 (-38.5, 18) -> (-33.5, 18)
  arc A65 (-33.5, 18) -> (-32.5, 19) centre (-33.5, 19) ccw
  line L182 (-32.5, 19) -> (-31, 19)
  line L183 (-31, 19) -> (-31, 9.5)
  line L184 (-31, 9.5) -> (-51.5, 9.5)
  line L185 (-51.5, 9.5) -> (-51.5, 5)
  circle A66 centre (-36, 14.5) radius 1.9
extrude "Extrusion40" add sketch "Skizze41" against normal blind 28 contours L61 A43 L62 L76 A46 L77 L90 A47 L91 L139 A52 L140 | A37 L48 A38 L135 L136 L173 L174 A63 L180 A64 | L56 A42 L57 L97 A49 L98 L144 A53 L145 | A39 L52 A40 L148 L149 L150 L158 A58 L165 A59 bodies 2
extrude "Extrusion41" cut 2 faces at (40.1667, 19, 15.3333) (40.1667, 19, -13.6667) along direction (0, 1, 0) blind 5.5 on bodies 2 bodies 2